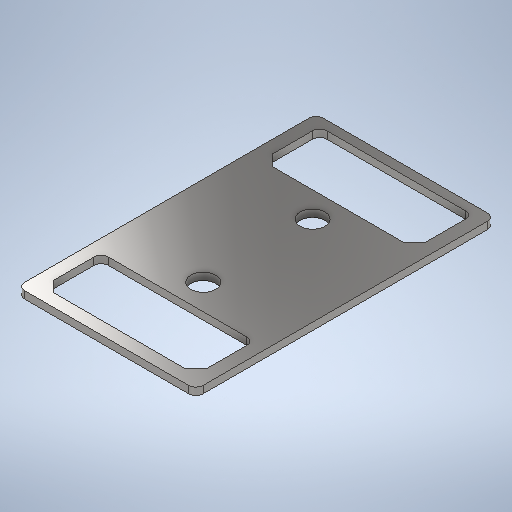
# Autodesk Inventor part: flex clamp V1
Saved by Autodesk Inventor 2025 (Build 290162000, 162)
## iProperties
Created: 2024-08-20
Part Number: flex clamp V1
Material: Stainless Steel
Document SubType Name: Modeling
Designer: Caleb Fangmeier
Density: 8 g/cm^3
Appearance: Semi-Polished
Author: Caleb Fangmeier
Autodesk Inventor part; units mm, degrees
ref_plane "YZ Plane" through (0, 0, 0) normal (1, 0, 0) x (0, 1, 0)
ref_plane "XZ Plane" through (0, 0, 0) normal (0, 1, 0) x (-1, 0, 0)
ref_plane "XY Plane" through (0, 0, 0) normal (0, 0, 1) x (1, 0, 0)
sketch "Sketch1" plane through (0, 0, 0) normal (0, 1, 0) x (-1, 0, 0)
  line L0 (-11.25, -20.5) -> (11.25, -20.5)
  line L1 (12.25, -19.5) -> (12.25, 19.5)
  line L2 (11.25, 20.5) -> (-11.25, 20.5)
  line L3 (-12.25, 19.5) -> (-12.25, -19.5)
  line L4 (-12.25, -20.5) -> (12.25, 20.5) construction
  line L5 (12.25, -20.5) -> (-12.25, 20.5) construction
  arc A0 (12.25, 19.5) -> (11.25, 20.5) centre (11.25, 19.5) ccw
  arc A1 (-11.25, 20.5) -> (-12.25, 19.5) centre (-11.25, 19.5) ccw
  arc A2 (-12.25, -19.5) -> (-11.25, -20.5) centre (-11.25, -19.5) ccw
  arc A3 (11.25, -20.5) -> (12.25, -19.5) centre (11.25, -19.5) ccw
  point P0 (0, 0)
  dimension "d0" = 24.5
  dimension "d1" = 41
  dimension "d2" = 1
  constraints: 12 end point, 8 point on circle, 8 point on line, 8 tangent, 4 centre point, 3 equal radius, 2 midpoint, 2 parallel, 1 horizontal, 1 perpendicular
  measures "d0" distance of L4.end L5.end
  measures "d1" distance of L5.start L4.end
  measures "d2" radius of A0
extrude "Extrusion1" add sketch "Sketch1" along normal blind 1
sketch "Sketch2" plane through (0, 1, 0) normal (0, 1, 0) x (1, 0, 0)
  line L0 (9.5, -10.75) -> (-9.5, -10.75)
  line L1 (-10.5, -11.75) -> (-10.5, -17.25)
  line L2 (-9, -18.75) -> (9, -18.75)
  line L3 (10.5, -17.25) -> (10.5, -11.75)
  line L4 (10.5, -10.75) -> (-10.5, -18.75) construction
  line L5 (-10.5, -10.75) -> (10.5, -18.75) construction
  line L6 (-9.5, 19.25) -> (9.5, 19.25)
  line L7 (10.5, 18.25) -> (10.5, 12.75)
  line L8 (9, 11.25) -> (-9, 11.25)
  line L9 (-10.5, 12.75) -> (-10.5, 18.25)
  line L10 (-10.5, 19.25) -> (10.5, 11.25) construction
  line L11 (10.5, 19.25) -> (-10.5, 11.25) construction
  line L12 (11.25, 20.5) -> (-11.25, 20.5) projected
  arc A0 (-9.5, -10.75) -> (-10.5, -11.75) centre (-9.5, -11.75) ccw
  arc A1 (10.5, -11.75) -> (9.5, -10.75) centre (9.5, -11.75) ccw
  arc A2 (-9.5, 19.25) -> (-10.5, 18.25) centre (-9.5, 18.25) ccw
  arc A3 (10.5, 18.25) -> (9.5, 19.25) centre (9.5, 18.25) ccw
  line L13 (10.5, -17.25) -> (9, -18.75)
  line L14 (10.5, 12.75) -> (9, 11.25)
  line L15 (-9, -18.75) -> (-10.5, -17.25)
  line L16 (-9, 11.25) -> (-10.5, 12.75)
  point P0 (0, 0)
  point P1 (0, -14.75)
  point P2 (0, 15.25)
  dimension "d5" = 30
  dimension "d8" = 1.25
  dimension "d9" = 8
  dimension "d10" = 8
  dimension "d11" = 21
  dimension "d12" = 21
  dimension "d14" = 1.5
  dimension "d15" = 1.5
  dimension "d16" = 1.5
  dimension "d17" = 1.5
  dimension "d18" = 1.5
  dimension "d19" = 1.5
  dimension "d20" = 1.5
  dimension "d21" = 1
  dimension "d22" = 1
  constraints: 32 end point, 16 point on line, 8 point on circle, 8 tangent, 5 parallel, 4 centre point, 4 midpoint, 2 equal radius, 2 horizontal, 2 perpendicular, 2 vertical alignment
  measures "d5" distance of point (0, 15.25) point (0, -14.75)
  measures "d8" distance between parallel lines of L12 L6
  measures "d9" distance of L11.end L10.start
  measures "d10" distance of L5.start L4.end
  measures "d11" distance of L10.end L11.end
  measures "d12" distance of L4.start L5.start
  measures "d14" horizontal distance of L3.start L2.end
  measures "d15" horizontal distance of L3.start L2.end
  measures "d16" horizontal distance of L7.end L8.start
  measures "d17" horizontal distance of L7.end L8.start
  measures "d18" horizontal distance of L2.start L1.end
  measures "d19" horizontal distance of L2.start L1.end
  measures "d20" horizontal distance of L8.end L9.start
  measures "d21" radius of A2
  measures "d22" radius of A0
extrude "Extrusion2" cut sketch "Sketch2" against normal through all
sketch "Sketch3" plane through (0, 1, 0) normal (0, 1, 0) x (1, 0, 0)
  line L0 (11.25, 20.5) -> (-11.25, 20.5) projected
  point P0 (0, 0)
  point P1 (0, -7.24)
  point P2 (0, 7.76)
  dimension "d23" = 15
  dimension "d24" = 12.74
  measures "d23" distance of point (0, -7.24) point (0, 7.76)
  measures "d24" distance from line of L0 point (0, 7.76)
hole "Hole1" at (0, 1, 7.24) at (0, 1, -7.76) direction (0, -1, 0) diameter 3.4 depth 7.9 tip angle 118 clearance for "Flat Head Machine Screw" size "M3" standard "Ansi Metric M Profile"
equation "\"d10\" = d9"
equation "\"d12\" = d11"
equation "\"d15\" = d14"
equation "\"d16\" = d14"
equation "\"d17\" = d15"
equation "\"d18\" = d15"
equation "\"d19\" = d14"
equation "\"d20\" = d15"
body "Solid1"
